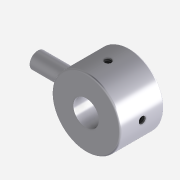
# Autodesk Inventor part: adapter
Saved by Autodesk Inventor 2018.2 (Build 222227000, 227)
## iProperties
Created: 2019-05-30
Part Number: adapter
Material: Generic
Document SubType Name: Modeling
Designer: Hannah Payne
Density: 1 g/cm^3
Appearance: Default
Author: Hannah Payne
Autodesk Inventor part; units mm, degrees
ref_plane "XZ Plane" through (0, 0, 0) normal (0, 1, 0) x (-1, 0, 0)
sketch "Sketch1" plane through (0, 0, 0) normal (0, 1, 0) x (-1, 0, 0)
  circle A0 centre (0, 0) radius 11
  dimension "d0" = 22
  constraints: 1 centre point, 1 coincident
  measures "d0" diameter of A0
extrude "Extrusion1" add sketch "Sketch1" along normal blind 14
sketch "Sketch2" plane through (0, 0, 0) normal (0, 1, 0) x (-1, 0, 0)
  point P0 (0, 0)
  point P1 (0, 0)
  constraints: 1 coincident
hole "Hole1" at (0, 0, 0) direction (0, 1, 0) diameter 8.2 end through all
ref_plane "Work Plane2" through (11, 0, 0) normal (1, 0, 0) x (0, 1, 0)
sketch "Sketch4" plane through (11, 0, 0) normal (1, 0, 0) x (0, 1, 0)
  line L0 (14, -11) -> (14, 11) construction
  line L1 (0, 0) -> (7, 0) construction
  line L2 (7, 0) -> (14, 0) construction
  constraints: 4 end point, 1 coincident, 1 collinear, 1 horizontal, 1 midpoint
hole "Hole2" at (11, 7, 0) direction (-1, 0, 0) diameter 2.156 end up to surface thread size "4-40 UNC" class "2B" standard "ANSI Unified Screw Threads"
pattern_circular "Circular Pattern1" count 3 over 180 about axis through (0, -10, 0) along (0, 1, 0) of "Hole2" both ways yes
shell "Shell2" thickness 1.5 removed faces 0
ref_plane "Work Plane1" through (-11, 0, 0) normal (1, 0, 0) x (0, 1, 0)
sketch "Sketch3" plane through (-11, 0, 0) normal (1, 0, 0) x (0, 1, 0)
  circle A0 centre (7, 0) radius 2.6
  line L0 (14, -11) -> (14, 11) construction
  line L1 (0, 11) -> (0, -11) construction
  line L2 (14, 0) -> (7, 0) construction
  line L3 (7, 0) -> (0, 0) construction
  dimension "d10" = 5.2
  constraints: 4 end point, 2 collinear, 1 centre point, 1 horizontal, 1 horizontal alignment, 1 midpoint
  measures "d10" diameter of A0
extrude "Extrusion2" add sketch "Sketch3" against normal blind 11.5 and the other way blind 1
fillet "Fillet1" radius 0.5 2 edges at (-10.6883, 7, -2.6) (-10.6883, 7, 2.6)
fillet "Fillet2" radius 0.5 2 edges at (11, 14, 0) (11, 0, 0)
body "Solid1"
